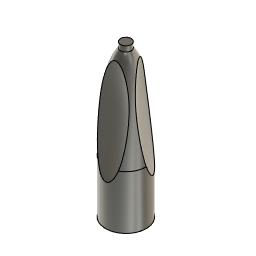
DEL_Speed (Autodesk Fusion 360 design; units mm, degrees)
Autodesk Fusion 360 part; units mm, degrees
sketch "スケッチ1" plane through (0, 0, 0) normal (0, 1, 0) x (1, 0, 0)
  line L0 (-9.5, 10) -> (-9.5, -15)
  line L1 (0, -68) -> (0, 11)
  spline S0 degree 5 poles (0, -60) (-0.3602, -59.9575) (-1.0769, -59.7463) (-2.1407, -59.0513) (-3.5201, -57.4041) (-5.0986, -54.3247) (-6.4456, -50.4266) (-7.5203, -45.8704) (-8.3285, -40.7565) (-8.8977, -35.1344) (-9.2657, -29.0097) (-9.4277, -23.6888) (-9.4869, -19.4453) (-9.5, -16.501) (-9.5, -15) knots 0 0 0 0 0 0 0.1 0.2 0.3 0.4 0.5 0.6 0.7 0.8 0.9 1 1 1 1 1 1
  line L2 (-9.5, -21.3) -> (-9.5, -8.7)
  line L3 (2.7818, -60.3284) -> (-2.7818, -59.6716)
  line L4 (-2.5, -60.9885) -> (-2.5, -58.4618)
  line L5 (-7.2, 10) -> (-9.5, 10)
  line L6 (-2.5, -60.9885) -> (0, -60.9885)
  line L7 (0, 0) -> (0, 10)
  line L8 (0, -55) -> (-1.4, -53.1333)
  line L9 (-3, -48.3333) -> (-3, 10)
  line L10 (-3, 10) -> (-9.5, 10)
  arc A0 (-3, -48.3333) -> (-1.4, -53.1333) centre (5, -48.3333) ccw
  point P0 (0, -30)
  point P1 (-9.5, -15)
  point P2 (0, -60)
  point P3 (0, 0)
  point P4 (0, -60)
  point P5 (-5.6023, -52.675)
  point P6 (0, -55)
  dimension "d10" = 25
  dimension "d14" = 9.5
  dimension "d16" = 60
  dimension "d25" = 5
  dimension "d30" = 70
  dimension "d51" = 8
  constraint vertical L1
  constraint coincident P1 L0.end
  constraint coincident L1 P4
  constraint coincident L1 P3
  constraint coincident P4 P2
  constraint midpoint P1 L2
  constraint coincident L0 L2.end
  constraint midpoint P4 L3
  constraint coincident S0 L4.end
  constraint coincident L1 P6
  constraint coincident L1 L6.end
  constraint perpendicular L1 L6
  constraint vertical L7
  constraint coincident L1 L7.end
  constraint coincident P6 L8.start
  constraint parallel L1 L9
  constraint tangent L8 A0
  constraint tangent L9 A0
  measures "d10" distance of L0.start P1
  measures "d14" distance of L0 L1
  measures "d16" distance of P4 P3
  measures "d25" distance of P4 P6
  measures "d30" distance of P4 L5
  measures "d51" radius of A0
revolve "回転2" add sketch "スケッチ1" angle 360 about axis through (0, 0, 68) along (0, 0, -1)
sketch "スケッチ5" plane through (0, 0, 60.9885) normal (0, 0, 1) x (-1, 0, 0)
  circle A0 centre (0, 0) radius 2.5
  point P0 (0, 0)
  constraint coincident P0 A0.centre
sketch "スケッチ6" plane through (0, 0, 60.9885) normal (0, 0, 1) x (-1, 0, 0)
  line L0 (0, 15) -> (0, 0)
  line L1 (0, 0) -> (-12.9904, -7.5)
  line L2 (0, 0) -> (12.9904, -7.5)
  line L3 (0, 0) -> (15, 0) construction
  point P0 (-6.4952, -3.75)
  point P1 (0, 7.5)
  point P2 (6.4952, -3.75)
  point P3 (0, 0)
  dimension "d31" = 120
  dimension "d32" = 15
  dimension "d33" = 30
  dimension "d34" = 15
  dimension "d35" = 7.5
  dimension "d36" = 7.5
  dimension "d37" = 7.5
  constraint coincident P3 L0.end
  constraint vertical L0
  constraint horizontal L3
  constraint midpoint L1 P0
  constraint midpoint L0 P1
  constraint coincident L2 P2
  measures "d31" angle of L0 L1
  measures "d32" distance of L0.end L1.end
  measures "d33" angle of L2 L3
  measures "d34" distance of P3 L2.end
  measures "d35" distance of P0 P3
  measures "d36" distance of P1 P3
  measures "d37" distance of P2 P3
ref_plane "作業平面1" through (0, 0, 0) normal (-0.5, 0.866025, 0) x (-0.866025, -0.5, 0)
sketch "スケッチ7" plane through (0, 0, 0) normal (-0.5, 0.866025, 0) x (-0.866025, -0.5, 0)
  line L0 (-15, 61) -> (-15, 0)
  line L1 (-5, 61) -> (-15, 0)
  spline S0 degree 5 poles (-5, 61) (-4.8728, 59.6806) (-4.6392, 57.0994) (-4.3517, 53.4006) (-4.0958, 48.8176) (-4.008, 43.6149) (-4.1866, 38.6502) (-4.6822, 33.3752) (-5.5542, 26.5246) (-6.8927, 18.4324) (-8.8062, 10.221) (-10.8877, 4.7397) (-12.8013, 1.8291) (-14.24, 0.5067) (-15, 0) knots 0 0 0 0 0 0 0.1 0.2 0.3 0.4 0.5 0.6 0.7 0.8 0.9 1 1 1 1 1 1
  line L2 (-4, 41) -> (-4.9933, 30.3825)
  line L3 (-12, 2) -> (-18, -2)
  line L4 (-25.26, 61.0426) -> (-35.26, 0.0426)
  point P0 (-4.4966, 35.6913)
  point P1 (0, 61)
  dimension "d40" = 20
  dimension "d43" = 5
  constraint vertical L0
  constraint midpoint P0 L2
  constraint midpoint L0.end L3
  constraint parallel L1 L4
  measures "d40" distance of L1 L4
  measures "d43" distance of L1.start P1
revolve "回転3" cut sketch "スケッチ7" angle 360 about axis through (21.8758, 12.63, 61.0426) along (0.140101, 0.080888, -0.986828)
ref_plane "作業平面2" through (0, 0, 0) normal (-1, 0, 0) x (0, -1, 0)
sketch "スケッチ8" plane through (0, 0, 0) normal (-1, 0, 0) x (0, 1, 0)
  line L0 (0, 0) -> (-50, 0)
  spline S0 degree 5 poles (-5, -61) (-4.8728, -59.6806) (-4.6392, -57.0994) (-4.3517, -53.4006) (-4.0958, -48.8176) (-4.008, -43.6149) (-4.1866, -38.6502) (-4.6822, -33.3752) (-5.5542, -26.5246) (-6.8927, -18.4324) (-8.8062, -10.221) (-10.8877, -4.7397) (-12.8013, -1.8291) (-14.24, -0.5067) (-15, 0) knots 0 0 0 0 0 0 0.1 0.2 0.3 0.4 0.5 0.6 0.7 0.8 0.9 1 1 1 1 1 1
  line L1 (-4, -41) -> (-4.9933, -30.3825)
  line L2 (-12, -2) -> (-18, 2)
  line L3 (-25.26, -61.0426) -> (-35.26, -0.0426)
  line L4 (-5, -61) -> (-15, 0)
  line L5 (-15, -61) -> (-15, 0)
  point P0 (-4.4966, -35.6913)
  point P1 (0, -61)
  dimension "d45" = 20
  dimension "d46" = 5
  constraint coincident L0.start origin
  constraint horizontal L0
  constraint midpoint P0 L1
  constraint midpoint S0.end L2
  constraint parallel L3 L4
  measures "d45" distance of L3 L4
  measures "d46" distance of S0.start P1
revolve "回転5" cut sketch "スケッチ8" angle 360 about axis through (0, -25.26, 61.0426) along (0, -0.161775, -0.986828)
ref_plane "作業平面3" through (0, 0, 0) normal (-0.5, -0.866025, 0) x (0.866025, -0.5, 0)
sketch "スケッチ9" plane through (0, 0, 0) normal (-0.5, -0.866025, 0) x (0.866025, -0.5, 0)
  spline S0 degree 5 poles (-5, 61) (-4.8728, 59.6806) (-4.6392, 57.0994) (-4.3517, 53.4006) (-4.0958, 48.8176) (-4.008, 43.6149) (-4.1866, 38.6502) (-4.6822, 33.3752) (-5.5542, 26.5246) (-6.8927, 18.4324) (-8.8062, 10.221) (-10.8877, 4.7397) (-12.8013, 1.8291) (-14.24, 0.5067) (-15, 0) knots 0 0 0 0 0 0 0.1 0.2 0.3 0.4 0.5 0.6 0.7 0.8 0.9 1 1 1 1 1 1
  line L0 (-4, 41) -> (-4.9933, 30.3825)
  line L1 (-12, 2) -> (-18, -2)
  line L2 (-25.26, 61.0426) -> (-35.26, 0.0426)
  line L3 (-5, 61) -> (-15, 0)
  line L4 (-15, 61) -> (-15, 0)
  point P0 (-4.4966, 35.6913)
  point P1 (0, 61)
  dimension "d48" = 20
  dimension "d49" = 5
  constraint vertical L4
  constraint midpoint P0 L0
  constraint midpoint S0.end L1
  constraint parallel L2 L3
  measures "d48" distance of L2 L3
  measures "d49" distance of S0.start P1
revolve "回転6" cut sketch "スケッチ9" angle 360 about axis through (-21.8758, 12.63, 61.0426) along (-0.140101, 0.080888, -0.986828)
hole "穴2" [rolled back] hole depth 10 hole diameter 1.3 tip angle 118
